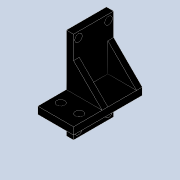
# Autodesk Inventor part: X Axis Limit Switch Bracket
Saved by Autodesk Inventor 2022 (Build 260153000, 153)
## iProperties
Created: 2021-10-25
Part Number: X Axis Limit Switch Bracket
Material: Generic
Document SubType Name: Modeling
Designer: Coy
Density: 1 g/cm^3
Appearance: Anodized - Black
Author: Coy
Autodesk Inventor part; units mm, degrees
ref_plane "YZ Plane" through (0, 0, 0) normal (1, 0, 0) x (0, 1, 0)
ref_plane "XZ Plane" through (0, 0, 0) normal (0, 1, 0) x (-1, 0, 0)
ref_plane "XY Plane" through (0, 0, 0) normal (0, 0, 1) x (1, 0, 0)
sketch "Sketch1" plane through (0, 0, 0) normal (1, 0, 0) x (0, 1, 0)
  line L0 (0, 0) -> (64, 0)
  line L1 (64, 0) -> (64, 28)
  line L2 (64, 28) -> (0, 28)
  line L3 (0, 28) -> (0, 0)
  line L4 (60, 24.5) -> (4, 24.5) construction
  line L5 (4, 24.5) -> (4, 3.5) construction
  line L6 (4, 3.5) -> (60, 3.5) construction
  line L7 (60, 3.5) -> (60, 24.5) construction
  line L8 (60, 24.5) -> (64, 24.5) construction
  line L9 (60, 24.5) -> (60, 28) construction
  line L10 (4, 3.5) -> (0, 3.5) construction
  line L11 (4, 3.5) -> (4, 0) construction
  circle A0 centre (60, 24.5) radius 2.6
  circle A1 centre (60, 3.5) radius 2.6
  circle A2 centre (4, 3.5) radius 2.6
  circle A3 centre (4, 24.5) radius 2.6
  dimension "d0" = 64
  dimension "d1" = 28
  dimension "d2" = 56
  dimension "d3" = 21
  dimension "d4" = 5.2
  dimension "d5" = 5.2
  dimension "d6" = 5.2
  dimension "d7" = 5.2
  constraints: 24 end point, 6 parallel, 6 perpendicular, 4 centre point, 4 coincident, 4 point on line, 2 horizontal
  measures "d0" distance of L2.end L1.end
  measures "d1" distance of L1.end L0.end
  measures "d2" distance of L6.end L5.end
  measures "d3" distance of L5.end L4.end
  measures "d4" diameter of A0
  measures "d5" diameter of A1
  measures "d6" diameter of A2
  measures "d7" diameter of A3
extrude "Extrusion1" add sketch "Sketch1" along normal blind 5
sketch "Sketch2" plane through (5, 0, 0) normal (1, 0, 0) x (0, 0, -1)
  line L0 (0, 0) -> (0, 64) projected
  line L1 (-28, 64) -> (-28, 0) projected
  line L2 (0, 23) -> (-28, 23)
  line L3 (-28, 23) -> (-28, 28)
  line L4 (-28, 28) -> (0, 28)
  line L5 (0, 28) -> (0, 23)
  line L6 (0, 64) -> (-28, 64) projected
  point P0 (0, 28)
  dimension "d10" = 41
  dimension "d11" = 5
  constraints: 8 end point, 2 parallel, 2 point on line, 1 horizontal, 1 perpendicular
  measures "d10" distance between parallel lines of L6 L2
  measures "d11" distance between parallel lines of L2 L4
extrude "Extrusion2" add sketch "Sketch2" along normal blind 20 contours L2 L1 L4 L0
sketch "Sketch3" plane through (0, 0, 28) normal (0, 0, 1) x (1, 0, 0)
  line L0 (5, 23) -> (25, 23) projected
  line L1 (0, 64) -> (0, 0) projected
  line L2 (25, 23) -> (0, 23)
  line L3 (0, 23) -> (0, 28)
  line L4 (0, 28) -> (25, 28)
  line L5 (25, 28) -> (25, 23)
  dimension "d14" = 5
  constraints: 8 end point, 2 parallel, 1 horizontal, 1 perpendicular, 1 point on line
  measures "d14" distance of L2.end L3.end
extrude "Extrusion3" add sketch "Sketch3" along normal blind 20
sketch "Sketch4" plane through (0, 28, 48) normal (0, 1, 0) x (1, 0, 0)
  line L0 (0, 20) -> (0, 0) construction
  line L1 (0, 10) -> (25, 10) construction
  line L2 (25, 20) -> (25, 0) construction
  circle A0 centre (6, 10) radius 2.75
  circle A1 centre (19, 10) radius 2.75
  point P0 (0, 48)
  dimension "d20" = 5.5
  dimension "d21" = 5.5
  dimension "d22" = 6
  dimension "d24" = 6
  constraints: 2 centre point, 2 end point, 2 midpoint, 2 point on line
  measures "d20" diameter of A0
  measures "d21" diameter of A1
  measures "d22" distance from line of L0 A0.centre
  measures "d24" distance from line of L2 A1.centre
extrude "Extrusion4" cut sketch "Sketch4" against normal up to next
sketch "Sketch7" plane through (5, 0, 0) normal (1, 0, 0) x (0, 0, -1)
  line L0 (-28, 28) -> (0, 28) projected
  line L1 (0, 28) -> (-4, 28)
  line L2 (-4, 28) -> (-4, 48)
  line L3 (-4, 48) -> (0, 48)
  line L4 (0, 48) -> (0, 28)
  line L5 (-28, 64) -> (-28, 28) projected
  line L6 (-28, 28) -> (-24, 28)
  line L7 (-24, 28) -> (-24, 48)
  line L8 (-24, 48) -> (-28, 48)
  line L9 (-28, 48) -> (-28, 28)
  point P0 (0, 0)
  dimension "d27" = 4
  dimension "d28" = 20
  dimension "d29" = 4
  constraints: 16 end point, 4 parallel, 2 horizontal, 2 perpendicular, 1 point on line
  measures "d27" distance of L2.end L3.end
  measures "d28" distance of L1.end L2.end
  measures "d29" distance of L8.end L7.end
extrude "Extrusion5" add sketch "Sketch7" along normal blind 20
chamfer "Chamfer2" distance 20 angle 45 2 edges at (25, 48, 2) (25, 48, 26)
equation "\"d5\" = d4"
equation "\"d6\" = d4"
equation "\"d7\" = d4"
equation "\"d24\" = d22"
body "Solid1"
